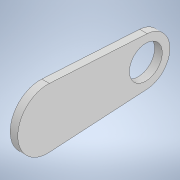
# Autodesk Inventor part: left_wall
Saved by Autodesk Inventor 2020 (Build 240168000, 168)
## iProperties
Created: 2024-02-19
Part Number: left_wall
Material: Типовые
Document SubType Name: Modeling
Designer: 4s
Density: 1 g/cm^3
Appearance: По умолчанию
Author: 4s
Autodesk Inventor part; units mm, degrees
ref_plane "YZ Plane" through (0, 0, 0) normal (1, 0, 0) x (0, 1, 0)
ref_plane "XZ Plane" through (0, 0, 0) normal (0, 1, 0) x (-1, 0, 0)
ref_plane "XY Plane" through (0, 0, 0) normal (0, 0, 1) x (1, 0, 0)
sketch "Эскиз1" plane through (0, 0, 0) normal (1, 0, 0) x (0, 1, 0)
  circle A0 centre (35.2311, -22.6062) radius 9.3
  circle A1 centre (0, -38.8201) radius 6.1
  circle A2 centre (0, 0) radius 4.85
  circle A3 centre (35.8147, -49.5529) radius 3.55
  line L0 (6.0968, -38.6237) -> (4.8475, 0.1562)
  line L1 (-4.8475, 0.1562) -> (-6.0968, -38.6237)
  line L2 (0, 0) -> (0, -38.8201) construction
  circle A4 centre (0, -38.8201) radius 6.5
  circle A5 centre (0, 0) radius 2
  circle A6 centre (0, -38.8201) radius 15 construction
  circle A7 centre (0, 0) radius 14 construction
  circle A8 centre (0, -38.8201) radius 9.5
  circle A9 centre (0, 0) radius 7
  line L3 (9.4833, -39.383) -> (11.7793, -0.6991)
  line L4 (-9.4833, -39.383) -> (-11.7793, -0.6991)
  circle A10 centre (0, 0) radius 8.8
  circle A11 centre (0, 0) radius 11.8
  point P0 (-7, 0)
  point P1 (-9.4833, -39.383)
  point P2 (-11.7793, -0.6991)
  dimension "d27" = 19
  dimension "d0" = 18.6
  dimension "d1" = 12.2
  dimension "d2" = 9.7
  dimension "d3" = 7.1
  dimension "d8" = 38.8201
  dimension "d13" = 38.8
  dimension "d14" = 38.8
  dimension "d23" = 13
  dimension "d24" = 4
  dimension "d25" = 30
  dimension "d26" = 28
  dimension "d28" = 14
  dimension "d31" = 17.6
  dimension "d32" = 3
  constraints: 10 centre point, 10 end point, 9 coincident, 4 point on circle, 4 tangent, 2 symmetric about line, 1 vertical, 8 other
  measures "d0" diameter of A0
  measures "d1" diameter of A1
  measures "d2" diameter of A2
  measures "d3" diameter of A3
  measures "d8" distance of L2.end L2.start
  measures "d13" distance of L0.start L0.end
  measures "d14" distance of L1.start L1.end
  measures "d23" diameter of A4
  measures "d24" diameter of A5
  measures "d25" diameter of A6
  measures "d26" diameter of A7
  measures "d28" diameter of A9
  measures "d31" diameter of A10
extrude "Выдавливание4" add sketch "Эскиз1" along normal blind 3 contours A4 L1 A8 L0 | L0 A8 L1 A4 | A8 L1 A11 L0 | L0 A11 L3 A8 | A8 L4 A11 L1 | A11 L1 A10 L0 | L0 A10 L1 A11 | A10 L1 A9 L0 | L0 A9 L1 A10 | A9 L1 A2 L0 | L0 A2 L1 A9 | A2 | A5
sketch "Эскиз4" plane through (0, 0, 0) normal (-1, 0, 0) x (0, 0, 1)
  circle A0 centre (-6.2, 6.2) radius 1.25
  circle A1 centre (-38.8201, 0) radius 6.5 construction
  arc A2 (-0.6991, -11.7793) -> (-0.6991, 11.7793) centre (0, 0) ccw construction
  line L0 (-39.383, 9.4833) -> (-0.6991, 11.7793) construction
  arc A3 (-39.383, 9.4833) -> (-39.383, -9.4833) centre (-38.8201, 0) ccw construction
  line L1 (-0.6991, -11.7793) -> (-39.383, -9.4833) construction
  line L2 (0, 0) -> (0, 11.8) construction
  arc A4 (-0.6991, -11.7793) -> (-0.6991, 11.7793) centre (0, 0) ccw construction
  line L3 (0, 0) -> (11.8, 0) construction
  circle A5 centre (6.2, 6.2) radius 1.25
  circle A6 centre (-6.2, -6.2) radius 1.25
  circle A7 centre (6.2, -6.2) radius 1.25
  dimension "d33" = 2.5
  dimension "d34" = 12.4
  dimension "d35" = 12.4
  constraints: 4 centre point, 4 end point, 3 point on circle, 3 symmetric about line, 1 vertical, 3 other
  measures "d33" diameter of A0
  measures "d34" distance of A5.centre A0.centre
  measures "d35" distance of A6.centre A0.centre
sketch "Эскиз5" plane through (3, 0, 0) normal (1, 0, 0) x (0, 0, -1)
  circle A0 centre (0, 0) radius 3.5
  dimension "d38" = 7
  constraints: 1 centre point, 1 coincident
  measures "d38" diameter of A0
